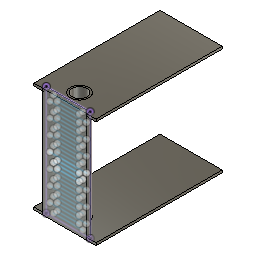
3ChamberBoxTube (Autodesk Fusion 360 design; units mm, degrees)
Autodesk Fusion 360 part; units mm, degrees
sketch "Door (1.25\" Tube)" plane through (0, 0, 0) normal (0, 0, 1) x (1, 0, 0)
  line L0 (0, 0) -> (107.95, 0)
  line L1 (107.95, 0) -> (107.95, 219.075)
  line L2 (107.95, 219.075) -> (0, 219.075)
  line L3 (0, 219.075) -> (0, 0)
  circle A0 centre (53.975, 25.4) radius 15.8115
  line L4 (15.875, 0) -> (15.875, 5.715)
  line L5 (15.875, 5.715) -> (92.075, 5.715)
  line L6 (92.075, 5.715) -> (92.075, 0)
  circle A1 centre (53.975, 25.4) radius 12.7
  dimension "d1" = 107.95
  dimension "d2" = 219.075
  dimension "d3" = 31.623
  dimension "d4" = 25.4
  dimension "d5" = 53.975
  dimension "d14" = 25.4
  dimension "d79" = 76.2
  dimension "d80" = 15.875
  dimension "d94" = 5.715
  constraint horizontal L0
  constraint vertical L1
  constraint horizontal L2
  constraint vertical L3
  constraint coincident L0.start L3.end
  constraint coincident L0 L4.start
  constraint perpendicular L0 L4
  constraint perpendicular L4 L5
  constraint perpendicular L5 L6
  constraint coincident L0 L6.end
  constraint concentric A0 A1
  measures "d1" distance of L0.start L0.end
  measures "d2" distance of L0.start L2.end
  measures "d3" diameter of A0
  measures "d4" distance of L0 A0.centre
  measures "d5" distance of L3 A0.centre
  measures "d14" diameter of A1
  measures "d79" distance of L4 L6
  measures "d80" distance of L1 L6
  measures "d94" distance of L0 L5
extrude "Extrude1" add sketch "Door (1.25\" Tube)" along normal blind 4.318 contours L0 L1 L2 L3 L4 L5 L6 makes body 1
extrude "Extrude2" add sketch "Door (1.25\" Tube)" along normal blind 4.318 separate body contours L0 L4 L5 L6 makes body 2
extrude "Extrude3" add sketch "Door (1.25\" Tube)" against normal blind 194.818 contours L0 L4 L5 L6 bodies 2
copy_body "CopyPasteBodies1" bodies 1 makes body 3
move_body "Move1" bodies 3 to x (1, 0, 0) y (0, 1, 0) z (0, 0, 1) at (0, 0, -194.818)
extrude "Extrude4" add sketch "Door (1.25\" Tube)" against normal up to surface (194.818 mm away) separate body contours A0 makes body 4
extrude "Extrude5" add 1 faces at (68.6432, 23.9835, 0) along direction (0, 0, 1) up to surface (4.318 mm away) on bodies 4 bodies 4
move_body "Move2" bodies 3 to x (1, 0, 0) y (0, 1, 0) z (0, 0, 1) at (0, 0, 8.636)
extrude "Extrude6" cut 1 faces at (66.675, 3.81, -194.818) along direction (0, 0, 1) blind 8.636 on bodies 2 bodies 2
extrude "Extrude7" cut 1 faces at (68.6432, 23.9835, -194.818) along direction (0, 0, 1) blind 8.636 on bodies 4 bodies 4
sketch "Tube Door Laser Cut" plane through (0, 0, 4.318) normal (0, 0, 1) x (-1, 0, 0)
  circle A0 centre (-53.975, -25.4) radius 15.8115
  line L0 (-92.075, -5.715) -> (-92.075, 0)
  line L1 (-92.075, 0) -> (-107.95, 0)
  line L2 (-107.95, 0) -> (-107.95, -219.075)
  line L3 (-107.95, -219.075) -> (0, -219.075)
  line L4 (0, -219.075) -> (0, 0)
  line L5 (0, 0) -> (-15.875, 0)
  line L6 (-15.875, 0) -> (-15.875, -5.715)
  line L7 (-15.875, -5.715) -> (-92.075, -5.715)
sketch "Base Laser Cut Engrave" plane through (0, 5.715, 0) normal (0, 1, 0) x (-1, 0, 0)
  line L0 (-92.075, -186.182) -> (-15.875, -186.182)
  line L1 (-15.875, -186.182) -> (-15.875, 4.318)
  line L2 (-15.875, 4.318) -> (-92.075, 4.318)
  line L3 (-92.075, 4.318) -> (-92.075, -186.182)
  line L4 (-22.225, -90.932) -> (-85.725, -90.932)
  line L5 (-34.925, -97.282) -> (-73.025, -97.282)
  line L6 (-28.575, -103.632) -> (-79.375, -103.632)
  line L7 (-34.925, -109.982) -> (-73.025, -109.982)
  line L8 (-22.225, -90.932) -> (-85.725, -90.932)
  line L9 (-34.925, -97.282) -> (-73.025, -97.282)
  line L10 (-28.575, -103.632) -> (-79.375, -103.632)
  line L11 (-34.925, -109.982) -> (-73.025, -109.982)
  line L12 (-22.225, -116.332) -> (-85.725, -116.332)
  line L13 (-34.925, -122.682) -> (-73.025, -122.682)
  line L14 (-28.575, -129.032) -> (-79.375, -129.032)
  line L15 (-34.925, -135.382) -> (-73.025, -135.382)
  line L16 (-22.225, -141.732) -> (-85.725, -141.732)
  line L17 (-34.925, -148.082) -> (-73.025, -148.082)
  line L18 (-28.575, -154.432) -> (-79.375, -154.432)
  line L19 (-34.925, -160.782) -> (-73.025, -160.782)
  line L20 (-22.225, -167.132) -> (-85.725, -167.132)
  line L21 (-34.925, -173.482) -> (-73.025, -173.482)
  line L22 (-28.575, -179.832) -> (-79.375, -179.832)
  line L23 (-34.925, -84.582) -> (-73.025, -84.582)
  line L24 (-28.575, -78.232) -> (-79.375, -78.232)
  line L25 (-34.925, -71.882) -> (-73.025, -71.882)
  line L26 (-22.225, -65.532) -> (-85.725, -65.532)
  line L27 (-34.925, -59.182) -> (-73.025, -59.182)
  line L28 (-28.575, -52.832) -> (-79.375, -52.832)
  line L29 (-34.925, -46.482) -> (-73.025, -46.482)
  line L30 (-22.225, -40.132) -> (-85.725, -40.132)
  line L31 (-34.925, -33.782) -> (-73.025, -33.782)
  line L32 (-28.575, -27.432) -> (-79.375, -27.432)
  line L33 (-34.925, -21.082) -> (-73.025, -21.082)
  line L34 (-22.225, -14.732) -> (-85.725, -14.732)
  line L35 (-34.925, -8.382) -> (-73.025, -8.382)
  line L36 (-28.575, -2.032) -> (-79.375, -2.032)
  dimension "d81" = 6.35
  dimension "d82" = 6.35
  dimension "d83" = 6.35
  dimension "d84" = 19.05
  dimension "d85" = 19.05
  dimension "d86" = 6.35
  dimension "d87" = 12.7
  dimension "d88" = 12.7
  dimension "d89" = 6.35
  dimension "d90" = 6.35
  dimension "d91" = 6.35
  dimension "d92" = 6.35
  dimension "d93" = 6.35
  constraint perpendicular L1 L4
  constraint horizontal L5
  constraint horizontal L6
  constraint horizontal L7
  constraint horizontal L9
  constraint horizontal L10
  constraint horizontal L11
  constraint horizontal L13
  constraint horizontal L14
  constraint horizontal L15
  constraint horizontal L17
  constraint horizontal L18
  constraint horizontal L19
  constraint horizontal L21
  constraint horizontal L22
  constraint symmetric L4 L6.end L24.end
  constraint symmetric L4 L6.start L24.start
  constraint symmetric L4 L5.start L23.start
  constraint symmetric L4 L5.end L23.end
  constraint symmetric L4 L7.start L25.start
  constraint symmetric L4 L7.end L25.end
  constraint symmetric L4 L12.end L26.end
  constraint symmetric L4 L12.start L26.start
  constraint symmetric L4 L14.end L28.end
  constraint symmetric L4 L14.start L28.start
  constraint symmetric L4 L13.start L27.start
  constraint symmetric L4 L13.end L27.end
  constraint symmetric L4 L15.start L29.start
  constraint symmetric L4 L15.end L29.end
  constraint symmetric L4 L16.start L30.start
  constraint symmetric L4 L16.end L30.end
  constraint symmetric L4 L18.end L32.end
  constraint symmetric L4 L18.start L32.start
  constraint symmetric L4 L19.start L33.start
  constraint symmetric L4 L17.start L31.start
  constraint symmetric L4 L17.end L31.end
  constraint symmetric L4 L19.end L33.end
  constraint symmetric L4 L22.end L36.end
  constraint symmetric L4 L22.start L36.start
  constraint symmetric L4 L21.end L35.end
  constraint symmetric L4 L20.start L34.start
  constraint symmetric L4 L20.end L34.end
  constraint symmetric L4 L21.start L35.start
  measures "d81" distance of L1 L4.start
  measures "d82" distance of L3 L4.end
  measures "d83" distance of L4 L5
  measures "d84" distance of L1 L5.start
  measures "d85" distance of L3 L5.end
  measures "d86" distance of L5 L6
  measures "d87" distance of L1 L6.start
  measures "d88" distance of L3 L6.end
  measures "d89" distance of L8 L9
  measures "d90" distance of L9 L10
  measures "d91" distance of L13 L14
  measures "d92" distance of L17 L18
  measures "d93" distance of L21 L22
sketch "Door (1.375\" Tube)" plane through (0, 0, 4.318) normal (0, 0, 1) x (-1, 0, 0)
  line L0 (-92.075, -5.715) -> (-92.075, 0)
  line L1 (-92.075, 0) -> (-107.95, 0)
  line L2 (-107.95, 0) -> (-107.95, -219.075)
  line L3 (-107.95, -219.075) -> (0, -219.075)
  line L4 (0, -219.075) -> (0, 0)
  line L5 (0, 0) -> (-15.875, 0)
  line L6 (-15.875, 0) -> (-15.875, -5.715)
  line L7 (-15.875, -5.715) -> (-92.075, -5.715)
  circle A0 centre (-53.975, -25.4) radius 17.4625
  dimension "d95" = 34.925
  measures "d95" diameter of A0
equation "d5 = ( 4.25 / 2 ) * 1 in"
equation "d12 = -7.5 in - 0.170 in"
named bodies: "Door 1", "Base Plate", "Door 2", "Tube"
